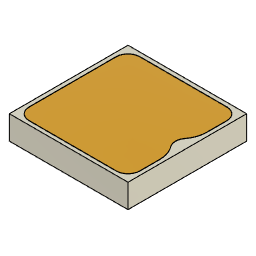
SunLike_LED_S1S0 (Autodesk Fusion 360 design; units mm, degrees)
Autodesk Fusion 360 part; units mm, degrees
note: some values were not read from the file. Set by a fixed rule: which sketch regions a step uses.
sketch "Sketch1" plane through (0, 0, 0) normal (0, 0, 1) x (1, 0, 0) in component "Body"
  line L0 (1.5, -1.5) -> (-1.5, -1.5)
  line L1 (-1.5, -1.5) -> (-1.5, 1.5)
  line L2 (-1.5, 1.5) -> (1.5, 1.5)
  line L3 (1.5, 1.5) -> (1.5, -1.5)
  line L4 (1.5, -1.5) -> (-1.5, 1.5) construction
  line L5 (-1.5, -1.5) -> (1.5, 1.5) construction
  dimension "d1" = 3
  dimension "d2" = 3
  constraint horizontal L0
  constraint perpendicular L0 L1
  constraint parallel L0 L2
  constraint parallel L1 L3
  constraint coincident L4 origin
  constraint coincident L5 origin
  measures "d1" distance of L1.end L2.end
  measures "d2" distance of L0.end L1.end
extrude "Extrude1" add sketch "Sketch1" along normal blind 0.6 makes body 1 in component "Body"
sketch "Sketch2" plane through (0, 0, 0.6) normal (0, 0, 1) x (-1, 0, 0) in component "Body"
  line L0 (-1.5, -1.5) -> (1.5, -1.5)
  line L1 (1.5, -1.5) -> (1.5, 1.5)
  line L2 (1.5, 1.5) -> (-1.5, 1.5)
  line L3 (-1.5, 1.5) -> (-1.5, -1.5)
  line L4 (-1.4, 1.4) -> (1.4, 1.4) construction
  line L5 (1.4, 1.4) -> (1.4, -1.4) construction
  line L6 (1.4, -1.4) -> (-1.4, -1.4) construction
  line L7 (-1.4, -1.4) -> (-1.4, 1.4) construction
  line L8 (-1.4, 1.4) -> (1.4, -1.4) construction
  line L9 (1.4, 1.4) -> (-1.4, -1.4) construction
  line L10 (1.4, 0) -> (-1.4, 0) construction
  arc A0 (1.1, -1.4) -> (1.4, -1.1) centre (1.1, -1.1) ccw
  line L11 (1.1, -1.1) -> (1.1, -1.4) construction
  line L12 (1.1, -1.1) -> (1.4, -1.1) construction
  arc A1 (-1.4, -1.1) -> (-1.1, -1.4) centre (-1.1, -1.1) ccw
  line L13 (-1.1, -1.1) -> (-1.4, -1.1) construction
  line L14 (-1.1, -1.1) -> (-1.1, -1.4) construction
  arc A2 (1.4, 1.1) -> (1.1, 1.4) centre (1.1, 1.1) ccw
  line L15 (1.1, 1.1) -> (1.4, 1.1) construction
  line L16 (1.1, 1.1) -> (1.1, 1.4) construction
  arc A3 (-1.1, 1.4) -> (-1.4, 1.1) centre (-1.1, 1.1) ccw
  line L17 (-1.1, 1.1) -> (-1.1, 1.4) construction
  line L18 (-1.1, 1.1) -> (-1.4, 1.1) construction
  line L19 (1.4, -1.1) -> (1.4, 1.1)
  line L20 (1.1, -1.4) -> (-1.1, -1.4)
  line L21 (1.1, 1.4) -> (-1.1, 1.4)
  line L22 (-1.4, 0) -> (-2.4, 0) construction
  line L23 (-1.4, -1.1) -> (-1.4, -1.0999)
  line L24 (-1.4, -1.0999) -> (-1.4, -0.5999)
  line L25 (-1.4, 1.1) -> (-1.4, 0.6)
  circle A4 centre (-1.5, 0) radius 0.3 construction
  arc A5 (-1.2543, -0.1721) -> (-1.2543, 0.1721) centre (-1.5, 0) ccw
  line L26 (-1.5, 0) -> (-1.2543, -0.1721) construction
  line L27 (-1.5, 0) -> (-1.2543, 0.1721) construction
  arc A6 (-1.2543, -0.1721) -> (-1.4, -0.5999) centre (-0.6989, -0.6) ccw
  arc A7 (-1.4, 0.6) -> (-1.2543, 0.1721) centre (-0.6989, 0.6) ccw
  dimension "d5" = 2.8
  dimension "d6" = 2.8
  dimension "d7" = 90
  dimension "d8" = 90
  dimension "d9" = 90
  dimension "d10" = 90
  dimension "d11" = 0.3
  dimension "d12" = 0.3
  dimension "d13" = 0.3
  dimension "d14" = 0.3
  dimension "d16" = 1
  dimension "d17" = 0.5
  dimension "d18" = 0.5
  dimension "d23" = 0.3
  dimension "d24" = 0.6
  dimension "d25" = 70
  constraint horizontal L4
  constraint perpendicular L4 L5
  constraint parallel L4 L6
  constraint parallel L5 L7
  constraint coincident L8 origin
  constraint coincident L9 origin
  constraint midpoint L5 L10.start
  constraint midpoint L7 L10.end
  constraint coincident L6 A0.start
  constraint coincident L8 A0.centre
  constraint coincident L6 A1.end
  constraint coincident L9 A1.centre
  constraint coincident L5 A2.start
  constraint coincident L9 A2.centre
  constraint coincident L7 A3.end
  constraint coincident L8 A3.centre
  constraint tangent L6 A0
  constraint tangent L6 A1
  constraint tangent L7 A3
  constraint tangent L4 A2
  constraint parallel L10 L22
  constraint coincident L7 L23.end
  constraint parallel L7 L24
  constraint perpendicular L18 L25
  constraint coincident L22 A4.centre
  constraint midpoint L3 A4.centre
  constraint coincident A4 A5.start
  constraint coincident A4.centre A5.centre
  constraint symmetric L10 A5.start A5.end
  constraint tangent L7 A6
  constraint tangent L7 A7
  constraint equal A6 A7
  measures "d5" distance of L5.end L6.end
  measures "d6" distance of L4.end L5.end
  measures "d7" angle of L11 L12
  measures "d8" angle of L13 L14
  measures "d9" angle of L15 L16
  measures "d10" angle of L17 L18
  measures "d11" distance of L5.end A0.start
  measures "d12" distance of L6.end A1.end
  measures "d13" distance of L4.end A2.end
  measures "d14" distance of L4.start A3.start
  measures "d16" distance of L10.end L22.end
  measures "d17" distance of L23.end L24.end
  measures "d18" distance of A3.end L25.end
  measures "d23" radius of A1
  measures "d24" diameter of A4
  measures "d25" angle of L26 L27
extrude "Extrude2" cut sketch "Sketch2" against normal blind 0.1 contours A0 A1 A2 A3 L19 L20 L21 L24 L25 A5 A6 A7 bodies 1 in component "Body"
sketch "Sketch3" plane through (0, 0, 0) normal (0, 0, -1) x (1, 0, 0) in component "Body"
  line L0 (-1.5, -1.5) -> (1.5, -1.5)
  line L1 (1.5, -1.5) -> (1.5, 1.5)
  line L2 (1.5, 1.5) -> (-1.5, 1.5)
  line L3 (-1.5, 1.5) -> (-1.5, -1.5)
  line L4 (-1.5, 0) -> (1.5, 0) construction
  line L5 (0.28, -1.09) -> (-1.25, -1.09) construction
  line L6 (-1.25, -1.09) -> (-1.25, 1.09) construction
  line L7 (-1.25, 1.09) -> (0.28, 1.09) construction
  line L8 (0.28, 1.09) -> (0.28, -1.09) construction
  line L9 (0.28, -1.09) -> (-1.25, 1.09) construction
  line L10 (-1.25, -1.09) -> (0.28, 1.09) construction
  line L11 (1.25, -1.09) -> (0.75, -1.09) construction
  line L12 (0.75, -1.09) -> (0.75, 1.09) construction
  line L13 (0.75, 1.09) -> (1.25, 1.09) construction
  line L14 (1.25, 1.09) -> (1.25, -1.09) construction
  line L15 (1.25, -1.09) -> (0.75, 1.09) construction
  line L16 (0.75, -1.09) -> (1.25, 1.09) construction
  line L17 (1.25, -1.09) -> (1.5, -1.09) construction
  line L18 (-1.25, -1.09) -> (-1.5, -1.09) construction
  arc A0 (1.25, 0.99) -> (1.15, 1.09) centre (1.15, 0.99) ccw
  line L19 (1.15, 0.99) -> (1.25, 0.99) construction
  line L20 (1.15, 0.99) -> (1.15, 1.09) construction
  arc A1 (0.85, 1.09) -> (0.75, 0.99) centre (0.85, 0.99) ccw
  line L21 (0.85, 0.99) -> (0.85, 1.09) construction
  line L22 (0.85, 0.99) -> (0.75, 0.99) construction
  arc A2 (1.15, -1.09) -> (1.25, -0.99) centre (1.15, -0.99) ccw
  line L23 (1.15, -0.99) -> (1.15, -1.09) construction
  line L24 (1.15, -0.99) -> (1.25, -0.99) construction
  arc A3 (0.75, -0.99) -> (0.85, -1.09) centre (0.85, -0.99) ccw
  line L25 (0.85, -0.99) -> (0.75, -0.99) construction
  line L26 (0.85, -0.99) -> (0.85, -1.09) construction
  arc A4 (0.18, -1.09) -> (0.28, -0.99) centre (0.18, -0.99) ccw
  line L27 (0.18, -0.99) -> (0.18, -1.09) construction
  line L28 (0.18, -0.99) -> (0.28, -0.99) construction
  arc A5 (0.28, 0.99) -> (0.18, 1.09) centre (0.18, 0.99) ccw
  line L29 (0.18, 0.99) -> (0.28, 0.99) construction
  line L30 (0.18, 0.99) -> (0.18, 1.09) construction
  line L31 (1.25, 0.99) -> (1.25, -0.99)
  line L32 (1.15, -1.09) -> (0.85, -1.09)
  line L33 (0.75, -0.99) -> (0.75, 0.99)
  line L34 (0.85, 1.09) -> (1.15, 1.09)
  line L35 (0.28, 0.99) -> (0.28, -0.99)
  line L36 (-1.25, 0.7) -> (-1.25, -0.7)
  arc A6 (-1.1803, 0.7953) -> (-1.25, 0.7) centre (-1.15, 0.7) ccw
  line L37 (-1.15, 0.7) -> (-1.1803, 0.7953) construction
  line L38 (-1.15, 0.7) -> (-1.25, 0.7) construction
  arc A7 (-1.25, -0.7) -> (-1.1803, -0.7953) centre (-1.15, -0.7) ccw
  line L39 (-1.15, -0.7) -> (-1.25, -0.7) construction
  line L40 (-1.15, -0.7) -> (-1.1803, -0.7953) construction
  arc A8 (-0.82, 1.09) -> (-0.9106, 1.0323) centre (-0.82, 0.99) ccw
  line L41 (-0.82, 0.99) -> (-0.82, 1.09) construction
  line L42 (-0.82, 0.99) -> (-0.9106, 1.0323) construction
  line L43 (0.18, 1.09) -> (-0.82, 1.09)
  line L44 (0.18, -1.09) -> (-0.82, -1.09)
  arc A9 (-0.9106, -1.0323) -> (-0.82, -1.09) centre (-0.82, -0.99) ccw
  line L45 (-0.82, -0.99) -> (-0.9106, -1.0323) construction
  line L46 (-0.82, -0.99) -> (-0.82, -1.09) construction
  arc A10 (-1.1803, 0.7953) -> (-0.9106, 1.0323) centre (-1.3155, 1.221) ccw
  arc A11 (-0.9106, -1.0323) -> (-1.1803, -0.7953) centre (-1.3155, -1.221) ccw
  point P0 (-0.485, 0)
  point P1 (1, 0)
  dimension "d28" = 1.53
  dimension "d29" = 2.18
  dimension "d30" = 0.5
  dimension "d31" = 2.18
  dimension "d32" = 0.47
  dimension "d33" = 90
  dimension "d34" = 90
  dimension "d35" = 90
  dimension "d36" = 90
  dimension "d37" = 90
  dimension "d38" = 90
  dimension "d39" = 0.1
  dimension "d43" = 65
  dimension "d45" = 0.1
  dimension "d46" = 1
  dimension "d47" = 1
  dimension "d48" = 65
  dimension "d49" = 0.1
  dimension "d50" = 1.4
  constraint midpoint L3 L4.start
  constraint midpoint L1 L4.end
  constraint horizontal L5
  constraint perpendicular L5 L6
  constraint parallel L5 L7
  constraint parallel L6 L8
  constraint coincident L9 P0
  constraint coincident L10 P0
  constraint coincident L4 P0
  constraint horizontal L11
  constraint perpendicular L11 L12
  constraint parallel L11 L13
  constraint parallel L12 L14
  constraint coincident L15 P1
  constraint coincident L16 P1
  constraint coincident L4 P1
  constraint coincident L1 L17.end
  constraint perpendicular L1 L17
  constraint coincident L3 L18.end
  constraint perpendicular L3 L18
  constraint equal L17 L18
  constraint coincident L13 A0.end
  constraint coincident L13 A1.start
  constraint coincident L14 A2.end
  constraint coincident L11 A3.end
  constraint coincident L8 A4.end
  constraint coincident L7 A5.end
  constraint tangent L8 A5
  constraint tangent L8 A4
  constraint tangent L12 A3
  constraint tangent L14 A2
  constraint tangent L14 A0
  constraint tangent L12 A1
  constraint tangent L13 A1
  constraint tangent L13 A0
  constraint tangent L11 A2
  constraint tangent L11 A3
  constraint tangent L5 A4
  constraint tangent L7 A5
  constraint equal A0 A1
  constraint equal A1 A5
  constraint equal A4 A5
  constraint equal A3 A4
  constraint equal A2 A3
  constraint coincident L6 L36.start
  constraint coincident L6 L36.end
  constraint symmetric L4 L36.start L36.end
  constraint tangent L6 A6
  constraint tangent L6 A7
  constraint equal A0 A6
  constraint equal A6 A7
  constraint coincident L7 A8.start
  constraint tangent L7 A8
  constraint perpendicular L30 L43
  constraint coincident A8.start L41.end
  constraint coincident L5 L44.end
  constraint perpendicular L27 L44
  constraint tangent L5 A9
  constraint tangent A8 A10
  constraint tangent A7 A11
  constraint tangent A9 A11
  constraint tangent A6 A10
  measures "d28" distance of L6.end L7.end
  measures "d29" distance of L5.end L6.end
  measures "d30" distance of L12.end L13.end
  measures "d31" distance of L11.end L12.end
  measures "d32" distance of L5.start L11.end
  measures "d33" angle of L19 L20
  measures "d34" angle of L21 L22
  measures "d35" angle of L23 L24
  measures "d36" angle of L25 L26
  measures "d37" angle of L27 L28
  measures "d38" angle of L29 L30
  measures "d39" radius of A0
  measures "d43" angle of L41 L42
  measures "d45" radius of A8
  measures "d46" distance of A5.end A8.start
  measures "d47" distance of A4.start L44.end
  measures "d48" angle of L45 L46
  measures "d49" radius of A9
  measures "d50" distance of L36.start L36.end
extrude "Extrude3" cut sketch "Sketch3" against normal blind 0.1 contours A0 A1 A2 A3 L31 L32 L33 L34 | A4 A5 L35 L36 A6 A7 A8 L43 L44 A9 A10 A11 bodies 1 in component "Body"
extrude "Extrude1'" add 1 faces at (-0.5331, 0.0068, 0.5) along direction (0, 0, 1) blind 0.095 separate body on bodies 1 makes body 2 in component "Element"
extrude "Extrude1''" add 2 faces at (-0.1535, 0.2952, 0.1) (1.0833, -0.33, 0.1) along direction (0, 0, -1) blind 0.11 separate body on bodies 1 makes body 3 at (-0.1535, 0.2952, 0.1) makes body 4 at (1.0833, -0.33, 0.1) in component "Pads"
component "Body" placed x (1, 0, 0) y (0, 1, 0) z (0, 0, 1) at (0, 0, 0)
component "Element" placed x (1, 0, 0) y (0, 1, 0) z (0, 0, 1) at (0, 0, 0)
component "Pads" placed x (1, 0, 0) y (0, 1, 0) z (0, 0, 1) at (0, 0, 0)
equation "d12 = d11"
equation "d13 = d11"
equation "d14 = d11"
equation "d45 = d39"
equation "d47 = d46"
equation "d49 = d45"
